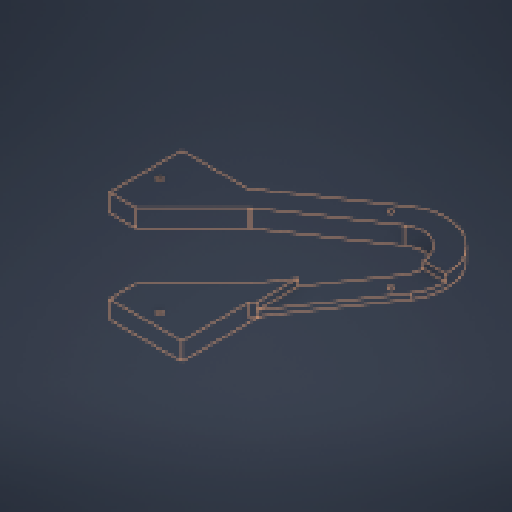
# Autodesk Inventor part: Front Right Cover Bracket
Saved by Autodesk Inventor 2023.1 (Build 271208000, 208)
## iProperties
Created: 2023-02-24
Part Number: Front Right Cover Bracket
Material: ABS Plastic
Document SubType Name: Modeling
Designer: remop
Density: 1.06 g/cm^3
Appearance: Smooth - Light Orange
Author: remop
Autodesk Inventor part; units mm, degrees
ref_plane "YZ Plane" through (0, 0, 0) normal (1, 0, 0) x (0, 1, 0)
ref_plane "XZ Plane" through (0, 0, 0) normal (0, 1, 0) x (-1, 0, 0)
ref_plane "XY Plane" through (0, 0, 0) normal (0, 0, 1) x (1, 0, 0)
sketch "Sketch13" plane through (0, 0, 0) normal (0, 0, 1) x (1, 0, 0)
  line L0 (-500, 9) -> (0, 9) construction
  line L1 (0, 9) -> (0, 15) projected
  line L2 (0, 15) -> (-500, 15) projected
  line L3 (-500, 9) -> (-500, 15) projected
  line L4 (6, 15) -> (6, 375) projected
  line L5 (0, 375) -> (6, 375) projected
  line L6 (0, 15) -> (0, 375) projected
  line L7 (0, 15) -> (6, 15) projected
  line L8 (-506, 375) -> (-506, 15) construction
  line L9 (-506, 15) -> (-500, 15) projected
  line L10 (-500, 15) -> (-500, 375) projected
  line L11 (-506, 375) -> (-500, 375) projected
  line L12 (-463.8988, 17.0711) -> (-473.7868, 17.0711) projected
  line L13 (-473.7868, 17.0711) -> (-497.9289, 41.2132) projected
  line L14 (-497.9289, 41.2132) -> (-497.9289, 51.1012) projected
  line L15 (-497.9289, 51.1012) -> (-466.8985, 82.1316) projected
  arc A0 (-466.4587, 82.4947) -> (-466.8985, 82.1316) centre (-464.7772, 80.0103) ccw projected
  line L16 (-466.4587, 82.4947) -> (-415.1076, 117.2506) projected
  arc A1 (-397.7494, 99.8924) -> (-415.1076, 117.2506) centre (-408.1012, 106.8988) ccw projected
  line L17 (-397.7494, 99.8924) -> (-432.5053, 48.5413) projected
  arc A2 (-432.8684, 48.1015) -> (-432.5053, 48.5413) centre (-434.9897, 50.2228) ccw projected
  line L18 (-432.8684, 48.1015) -> (-463.8988, 17.0711) projected
  circle A3 centre (-460.0736, 33.7132) radius 4 projected
  circle A4 centre (-438.8604, 54.9264) radius 4 projected
  circle A5 centre (-460.0736, 76.1396) radius 4 projected
  circle A6 centre (-481.2868, 54.9264) radius 4 projected
  circle A7 centre (-460.0736, 54.9264) radius 13 projected
  line L19 (-430.7901, 47.3804) -> (-396.0343, 98.7315)
  arc A8 (-396.0343, 98.7315) -> (-416.2685, 118.9657) centre (-408.1012, 106.8988) ccw
  line L20 (-416.2685, 118.9657) -> (-467.6196, 84.2099)
  arc A9 (-467.6196, 84.2099) -> (-468.363, 83.5961) centre (-464.7772, 80.0103) ccw
  line L21 (-468.363, 83.5961) -> (-500, 51.9591)
  line L22 (-500, 51.9591) -> (-500, 40.3553)
  line L23 (-500, 40.3553) -> (-474.6447, 15)
  line L24 (-474.6447, 15) -> (-463.0409, 15)
  line L25 (-463.0409, 15) -> (-431.4039, 46.637)
  arc A10 (-431.4039, 46.637) -> (-430.7901, 47.3804) centre (-434.9897, 50.2228) ccw
  line L26 (-385.3272, 91.4847) -> (-420.0831, 40.1336)
  arc A11 (-422.2618, 37.4949) -> (-420.0831, 40.1336) centre (-434.9897, 50.2228) ccw
  line L27 (-422.2618, 37.4949) -> (-457.6856, 2.0711)
  line L28 (-457.6856, 2.0711) -> (-480, 2.0711)
  line L29 (-480, 2.0711) -> (-512.9289, 35)
  line L30 (-512.9289, 35) -> (-512.9289, 57.3144)
  line L31 (-512.9289, 57.3144) -> (-477.5051, 92.7382)
  arc A12 (-474.8664, 94.9169) -> (-477.5051, 92.7382) centre (-464.7772, 80.0103) ccw
  line L32 (-474.8664, 94.9169) -> (-423.5153, 129.6728)
  arc A13 (-385.3272, 91.4847) -> (-423.5153, 129.6728) centre (-408.1012, 106.8988) ccw
  line L33 (-422.2618, 37.4949) -> (-422.2618, 0)
  line L34 (-477.5051, 92.7382) -> (-515, 92.7382)
  line L35 (0, 6) -> (-500, 6) construction
  line L36 (-500, 0) -> (-500, 6) projected
  line L37 (0, 0) -> (-500, 0) projected
  line L38 (0, 0) -> (0, 6) projected
  line L39 (-509, 15) -> (-509, 375) construction
  line L40 (-515, 375) -> (-509, 375) projected
  line L41 (-515, 15) -> (-515, 375) projected
  line L42 (-515, 15) -> (-509, 15) projected
  line L43 (-500, 51.9591) -> (-515, 51.9591)
  line L44 (-463.0409, 15) -> (-463.0409, 0)
  point P0 (-422.2618, 15)
  point P1 (-500, 92.7382)
  dimension "d27" = 15
  constraints: 36 end point, 13 point on circle, 10 point on line, 6 centre point, 4 perpendicular, 3 coincident, 2 horizontal alignment, 18 other
  measures "d27" distance between parallel lines of L17 L26
extrude "Extrusion14" add sketch "Sketch13" along normal blind 10 contours L25 A10 L19 A8 L20 A9 L21 L10 L31 A12 L32 A13 L26 A11 L27 L2 | L2 L27 L28 L44 | L27 L33 L2 | L2 L33 L37 L44 L28 L27 | L43 L30 L31 L10 | L31 L30 L43 L41 L34 L10 | L10 L34 L31
sketch "Sketch14" plane through (0, 0, 0) normal (0, 0, -1) x (-1, 0, 0)
  line L0 (467.6196, 84.2099) -> (416.2685, 118.9657) projected
  arc A0 (468.363, 83.5961) -> (467.6196, 84.2099) centre (464.7772, 80.0103) ccw projected
  line L1 (500, 51.9591) -> (468.363, 83.5961) projected
  line L2 (515, 51.9591) -> (500, 51.9591) projected
  line L3 (515, 92.7382) -> (515, 51.9591) projected
  line L4 (477.5051, 92.7382) -> (515, 92.7382) projected
  arc A1 (477.5051, 92.7382) -> (474.8664, 94.9169) centre (464.7772, 80.0103) ccw projected
  line L5 (423.5153, 129.6728) -> (474.8664, 94.9169) projected
  arc A2 (423.5153, 129.6728) -> (385.3272, 91.4847) centre (408.1012, 106.8988) ccw projected
  line L6 (420.0831, 40.1336) -> (385.3272, 91.4847) projected
  arc A3 (420.0831, 40.1336) -> (422.2618, 37.4949) centre (434.9897, 50.2228) ccw projected
  line L7 (422.2618, 0) -> (422.2618, 37.4949) projected
  line L8 (463.0409, 0) -> (422.2618, 0) projected
  line L9 (463.0409, 15) -> (463.0409, 0) projected
  line L10 (431.4039, 46.637) -> (463.0409, 15) projected
  arc A4 (430.7901, 47.3804) -> (431.4039, 46.637) centre (434.9897, 50.2228) ccw projected
  line L11 (396.0343, 98.7315) -> (430.7901, 47.3804) projected
  arc A5 (416.2685, 118.9657) -> (396.0343, 98.7315) centre (408.1012, 106.8988) ccw projected
  arc A6 (421.8736, 127.2472) -> (387.7528, 93.1264) centre (408.1012, 106.8988) ccw
  line L12 (421.8736, 127.2472) -> (473.2247, 92.4914)
  arc A7 (476.2278, 89.8093) -> (473.2247, 92.4914) centre (464.7772, 80.0103) ccw
  line L13 (476.2278, 89.8093) -> (512.0711, 89.8093)
  line L14 (512.0711, 89.8093) -> (512.0711, 54.888)
  line L15 (512.0711, 54.888) -> (501.2132, 54.888)
  line L16 (501.2132, 54.888) -> (470.434, 85.6672)
  arc A8 (470.434, 85.6672) -> (469.2613, 86.6355) centre (464.7772, 80.0103) ccw
  line L17 (469.2613, 86.6355) -> (417.9102, 121.3913)
  arc A9 (417.9102, 121.3913) -> (393.6087, 97.0898) centre (408.1012, 106.8988) ccw
  line L18 (393.6087, 97.0898) -> (428.3645, 45.7387)
  arc A10 (428.3645, 45.7387) -> (429.3328, 44.566) centre (434.9897, 50.2228) ccw
  line L19 (429.3328, 44.566) -> (460.112, 13.7868)
  line L20 (460.112, 13.7868) -> (460.112, 2.9289)
  line L21 (460.112, 2.9289) -> (425.1907, 2.9289)
  line L22 (425.1907, 2.9289) -> (425.1907, 38.7722)
  arc A11 (422.5086, 41.7753) -> (425.1907, 38.7722) centre (434.9897, 50.2228) ccw
  line L23 (422.5086, 41.7753) -> (387.7528, 93.1264)
  line L24 (422.2618, 0) -> (422.2618, 37.4949) projected
  line L25 (422.2618, 37.4949) -> (422.2618, 54.7554)
  line L26 (477.5051, 92.7382) -> (515, 92.7382) projected
  line L27 (477.5051, 92.7382) -> (455.0191, 92.7382)
  line L28 (467.6196, 84.2099) -> (416.2685, 118.9657) projected
  point P0 (0, 0)
  point P1 (460.2446, 92.7382)
  dimension "d32" = 10
  constraints: 28 end point, 12 point on circle, 6 centre point, 2 point on line, 1 collinear, 1 perpendicular, 17 other
  measures "d32" distance between parallel lines of L6 L18
extrude "Extrusion15" cut sketch "Sketch14" against normal blind 3 contours L17 A9 L18 L25 L23 A6 L12 L27 | L12 A6 L23 L25 A3 L6 A2 L5 A1 L27
sketch "Sketch15" plane through (0, 0, 10) normal (0, 0, 1) x (1, 0, 0)
  line L0 (-467.6196, 84.2099) -> (-416.2685, 118.9657) projected
  arc A0 (-396.0343, 98.7315) -> (-416.2685, 118.9657) centre (-408.1012, 106.8988) ccw projected
  line L1 (-396.0343, 98.7315) -> (-430.7901, 47.3804) projected
  arc A1 (-431.4039, 46.637) -> (-430.7901, 47.3804) centre (-434.9897, 50.2228) ccw projected
  line L2 (-431.4039, 46.637) -> (-463.0409, 15) projected
  line L3 (-463.0409, 15) -> (-463.0409, 0) projected
  line L4 (-463.0409, 0) -> (-422.2618, 0) projected
  line L5 (-422.2618, 0) -> (-422.2618, 37.4949) projected
  arc A2 (-422.2618, 37.4949) -> (-420.0831, 40.1336) centre (-434.9897, 50.2228) ccw projected
  line L6 (-420.0831, 40.1336) -> (-385.3272, 91.4847) projected
  arc A3 (-385.3272, 91.4847) -> (-423.5153, 129.6728) centre (-408.1012, 106.8988) ccw projected
  line L7 (-423.5153, 129.6728) -> (-474.8664, 94.9169) projected
  arc A4 (-474.8664, 94.9169) -> (-477.5051, 92.7382) centre (-464.7772, 80.0103) ccw projected
  line L8 (-477.5051, 92.7382) -> (-515, 92.7382) projected
  line L9 (-515, 92.7382) -> (-515, 51.9591) projected
  line L10 (-515, 51.9591) -> (-500, 51.9591) projected
  line L11 (-500, 51.9591) -> (-468.363, 83.5961) projected
  arc A5 (-467.6196, 84.2099) -> (-468.363, 83.5961) centre (-464.7772, 80.0103) ccw projected
  line L12 (-396.0343, 98.7315) -> (-430.7901, 47.3804) projected
  line L13 (-420.0831, 40.1336) -> (-385.3272, 91.4847) projected
  line L14 (-420.0831, 63.1999) -> (-420.0831, 40.1336)
  arc A6 (-396.0343, 98.7315) -> (-416.2685, 118.9657) centre (-408.1012, 106.8988) ccw projected
  line L15 (-393.5302, 106.8988) -> (-380.6012, 106.8988)
  arc A7 (-385.3272, 91.4847) -> (-423.5153, 129.6728) centre (-408.1012, 106.8988) ccw projected
  point P0 (0, 0)
  constraints: 4 end point, 2 point on circle, 1 horizontal, 1 horizontal alignment, 1 point on line, 1 vertical
extrude "Extrusion16" cut sketch "Sketch15" against normal blind 4 contours L15 A3 L6 L14 L1 A0
sketch "Sketch16" plane through (0, 0, 3) normal (0, 0, -1) x (-1, 0, 0)
  line L0 (420.0831, 40.1336) -> (385.3272, 91.4847) projected
  arc A0 (423.5153, 129.6728) -> (385.3272, 91.4847) centre (408.1012, 106.8988) ccw projected
  line L1 (423.5153, 129.6728) -> (474.8664, 94.9169) projected
  point P0 (0, 0)
  point P1 (393.3272, 88.4847)
  point P2 (426.5153, 121.6728)
  dimension "d37" = 8
  dimension "d38" = 3
  dimension "d39" = 8
  dimension "d40" = 3
  measures "d37" horizontal distance of L0.end point (393.327, 88.485)
  measures "d38" vertical distance of L0.end point (393.327, 88.485)
  measures "d39" vertical distance of L1.start point (426.515, 121.673)
  measures "d40" horizontal distance of L1.start point (426.515, 121.673)
hole "Hole1" at (-393.3272, 88.4847, 3) at (-426.5153, 121.6728, 3) direction (0, 0, 1) diameter 2.9 end through all
sketch "Sketch17" plane through (0, 0, 10) normal (0, 0, 1) x (1, 0, 0)
  line L0 (-422.2618, 0) -> (-422.2618, 37.4949) projected
  line L1 (-477.5051, 92.7382) -> (-515, 92.7382) projected
  point P0 (0, 0)
  point P1 (-442.2618, 7.5)
  point P2 (-507.5, 72.7382)
  point P3 (-422.2618, 18.7474)
  dimension "d48" = 7.5
  dimension "d49" = 7.5
  dimension "d50" = 20
  dimension "d51" = 20
  constraints: 1 midpoint
  measures "d48" horizontal distance of L1.end point (-507.5, 72.738)
  measures "d49" vertical distance of L0.start point (-442.262, 7.5)
  measures "d50" horizontal distance of point (-422.262, 18.747) point (-442.262, 7.5)
  measures "d51" distance from line of L1 point (-507.5, 72.738)
hole "Hole2" at (-442.2618, 7.5, 10) at (-507.5, 72.7382, 10) direction (0, 0, -1) diameter 3.2 end through all
equation "\"d40\" = d38"
equation "\"d49\" = d48"
equation "\"d51\" = d50"
body "Solid11"
